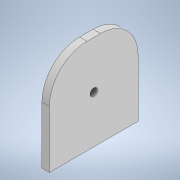
# Autodesk Inventor part: Base_Attachment
Saved by Autodesk Inventor 2022 (Build 260153000, 153)
## iProperties
Created: 2022-01-01
Part Number: Base_Attachment
Material: Generic
Document SubType Name: Modeling
Designer: Mlees
Density: 1 g/cm^3
Appearance: Default
Author: Mlees
Autodesk Inventor part; units mm, degrees
ref_plane "YZ Plane" through (0, 0, 0) normal (1, 0, 0) x (0, 1, 0)
ref_plane "XZ Plane" through (0, 0, 0) normal (0, 1, 0) x (-1, 0, 0)
ref_plane "XY Plane" through (0, 0, 0) normal (0, 0, 1) x (1, 0, 0)
sketch "Sketch1" plane through (0, 0, 0) normal (1, 0, 0) x (0, 1, 0)
  line L0 (0, 0) -> (101.6, 0)
  line L1 (101.6, 0) -> (101.6, -94.996)
  line L2 (101.6, -94.996) -> (0, -94.996)
  line L3 (0, -94.996) -> (0, 0)
  dimension "d0" = 101.6
  dimension "d1" = 94.996
  constraints: 8 end point, 2 parallel, 1 horizontal, 1 perpendicular
  measures "d0" distance of L1.end L2.end
  measures "d1" distance of L0.end L1.end
extrude "Extrusion1" add sketch "Sketch1" along normal blind 8
sketch "Sketch2" plane through (0, 0, -94.996) normal (0, -1, 0) x (1, 0, 0)
  line L0 (0, 0) -> (0, 94.996) projected
  line L1 (8, 0) -> (8, 94.996) projected
  circle A0 centre (4, 72.498) radius 2
  circle A1 centre (4, 22.498) radius 2
  dimension "d6" = 4
  constraints: 2 centre point
  measures "d6" diameter of A0
extrude "Extrusion2" cut sketch "Sketch2" against normal blind 8
sketch "Sketch3" plane through (8, 0, 0) normal (1, 0, 0) x (0, 0, -1)
  line L0 (0, 101.6) -> (0, 0) projected
  line L1 (94.996, 101.6) -> (0, 101.6) projected
  circle A0 centre (47.498, 50.8) radius 4
  dimension "d9" = 8
  constraints: 1 centre point
  measures "d9" diameter of A0
extrude "Extrusion3" cut sketch "Sketch3" against normal through all
fillet "Fillet1" radius 40.25 2 edges at (4, 101.6, 0) (4, 101.6, -94.996)
body "Solid1"
